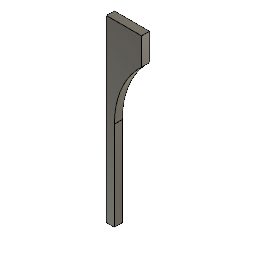
Retainer key (Autodesk Fusion 360 design; units mm, degrees)
Autodesk Fusion 360 part; units mm, degrees
sketch "Sketch1" plane through (0, 0, 0) normal (0, 0, 1) x (1, 0, 0)
  line L0 (2.25, 2.25) -> (-2.25, 2.25)
  line L1 (-2.25, 2.25) -> (-2.25, -2.25)
  line L2 (-2.25, -2.25) -> (2.25, -2.25)
  line L3 (2.25, -2.25) -> (2.25, 2.25)
  line L4 (2.25, 2.25) -> (-2.25, -2.25) construction
  line L5 (-2.25, 2.25) -> (2.25, -2.25) construction
  dimension "d1" = 4.5
  dimension "d2" = 4.5
extrude "Extrude1" add sketch "Sketch1" along normal blind 100
sketch "Sketch2" plane through (2.25, 0, 0) normal (1, 0, 0) x (0, 1, 0)
  line L0 (-2.25, 0) -> (2.25, 0)
  line L1 (2.25, 0) -> (2.25, 100)
  line L2 (2.25, 100) -> (-2.25, 100)
  line L3 (-2.25, 100) -> (-2.25, 0)
  line L4 (-2.25, 84.9965) -> (2.25, 84.9965)
extrude "Extrude2" add sketch "Sketch2" along normal blind 15 contours L1 L2 L3 L4
fillet "Fillet1" radius 47.5 1 edges at (2.25, 0, 84.9965)
chamfer "Chamfer1" distance 1 angle 45 4 edges at (2.25, 0, 0) (0, 2.25, 0) (0, -2.25, 0) (-2.25, 0, 0)
